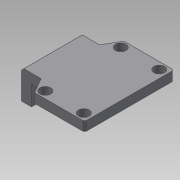
# Autodesk Inventor part: Крышка 6
Saved by Autodesk Inventor 2014 SP1 (Build 180222100, 222)
## iProperties
Created: 2021-12-02
Part Number: Крышка 6
Material: Типовые
Document SubType Name: Modeling
Designer: Украинцев
Mass: 144.48 g
Surface Area: 324.791 cm^2
Volume: 144.48 cm^3
Density: 1 g/cm^3
Appearance: По умолчанию
Author: Украинцев
Autodesk Inventor part; units mm, degrees
ref_plane "YZ Plane" through (0, 0, 0) normal (1, 0, 0) x (0, 1, 0)
ref_plane "XZ Plane" through (0, 0, 0) normal (0, 1, 0) x (-1, 0, 0)
ref_plane "XY Plane" through (0, 0, 0) normal (0, 0, 1) x (1, 0, 0)
sketch "Эскиз1" plane through (0, 0, 0) normal (0, 0, 1) x (1, 0, 0)
  line L0 (0, 0) -> (0, 58)
  line L1 (0, 58) -> (-65, 58)
  line L2 (-65, 58) -> (-76.547, 38)
  line L3 (-76.547, 38) -> (-102, 38)
  line L4 (-102, 38) -> (-102, 0)
  line L5 (-102, 0) -> (0, 0)
  line L6 (-89, 38) -> (-89, 0)
  point P0 (-60, 49)
  point P1 (-10, 49)
  dimension "d0" = 116
  dimension "d1" = 76
  dimension "d2" = 60
  dimension "d3" = 65
  dimension "d4" = 102
  dimension "d5" = 13
  dimension "d6" = 50
  dimension "d7" = 10
  dimension "d8" = 98
  constraints: 14 end point, 3 parallel, 2 perpendicular, 2 point on line, 1 horizontal alignment, 1 vertical
  measures "d0" diameter of L1 L5
  measures "d1" diameter of L3 L5
  measures "d2" angle of L1 L2
  measures "d3" distance of L0.end L1.end
  measures "d4" distance of L4.end L0.start
  measures "d5" distance between parallel lines of L6 L4
  measures "d6" distance of point (-10, 49) point (-60, 49)
  measures "d7" distance from line of L0 point (-10, 49)
  measures "d8" diameter of point (-10, 49) L5
extrude "Выдавливание1" add sketch "Эскиз1" against normal blind 12 contours L5 L6 L3 L2 L1 L0
extrude "Выдавливание2" add sketch "Эскиз1" against normal blind 38 contours L5 L4 L3 L6
hole "Отверстие1" at (-60, 49, 0) at (-10, 49, 0) direction (0, 0, -1) diameter 9 end through all counterbore diameter 14 counterbore depth 9
hole "Отверстие2" at (-102, 28, -27) direction (1, 0, 0) diameter 8.376 end through all thread size "M10x1.5" class "6H" standard "ISO Metric profile"
chamfer "Фаска1" distance 1.6 angle 45 1 edges at (-102, 28, -31.188)
chamfer "Фаска2" distance 3 angle 45 1 edges at (-102, 19, 0)
chamfer "Фаска3" distance 2 angle 45 1 edges at (0, 58, -6)
mirror "Зеркальное отражение1" about plane through (0, 0, 0) normal (0, -1, 0)
